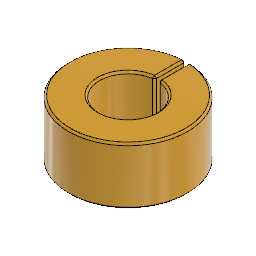
Z_limit_ring v1 (Autodesk Fusion 360 design; units mm, degrees)
Autodesk Fusion 360 part; units mm, degrees
sketch "Sketch1" plane through (0, 0, 0) normal (0, 0, 1) x (1, 0, 0)
  circle A0 centre (0, 0) radius 12.5
  circle A1 centre (0, 0) radius 6
  line L0 (0, -12.5) -> (0, 12.5) construction
  line L1 (-0.4, 12.5) -> (0.4, 12.5)
  line L2 (0.4, 12.5) -> (0.4, 0)
  line L3 (0.4, 0) -> (-0.4, 0)
  line L4 (-0.4, 0) -> (-0.4, 12.5)
  dimension "d1" = 25
  dimension "d2" = 12
  dimension "d3" = 0.8
  constraint coincident A0.centre A1.centre
  constraint concentric A0 A1
  constraint coincident A0 L0.start
  constraint coincident A0 L0.end
  constraint vertical L0
  constraint horizontal L1
  constraint vertical L2
  constraint horizontal L3
  constraint vertical L4
  constraint tangent A0 L1
  constraint midpoint L0.end L1
  measures "d1" diameter of A0
  measures "d2" diameter of A1
  measures "d3" distance of L2 L4
extrude "Extrude1" add sketch "Sketch1" along normal blind 12 contours A0 A1 L2 L4 picked at (-10.2052, -1.474)
chamfer "Chamfer1" distance 0.4 angle 45 12 edges at (0, -6, 0) (0, -12.5, 0) (0, -6, 12) (0, -12.5, 12) (0.4, 9.2401, 0) (0.4, 9.2401, 12) (-0.4, 9.2401, 0) (-0.4, 9.2401, 12) (0.4, 5.9867, 6) (-0.4, 5.9867, 6) (0.4, 12.4936, 6) (-0.4, 12.4936, 6)
